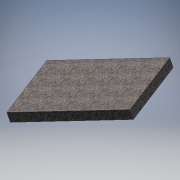
# Autodesk Inventor part: BaseMini
Saved by Autodesk Inventor 2016 (Build 200138000, 138)
## iProperties
Created: 2015-08-01
Part Number: BaseMini
Material: Concrete
Document SubType Name: Modeling
Designer: myhome
Density: 2.40731 g/cm^3
Appearance: Exposed Aggregate - Coarse
Mass: 231102 g
Surface Area: 23200 cm^2
Volume: 96000 cm^3
Author: myhome
Autodesk Inventor part; units mm, degrees
ref_plane "YZ Plane" through (0, 0, 0) normal (1, 0, 0) x (0, 1, 0)
ref_plane "XZ Plane" through (0, 0, 0) normal (0, 1, 0) x (-1, 0, 0)
ref_plane "XY Plane" through (0, 0, 0) normal (0, 0, 1) x (1, 0, 0)
sketch "Sketch5" plane through (0, 0, 0) normal (0, 0, 1) x (1, 0, 0)
  line L0 (0, 0) -> (1200, 0)
  line L1 (1200, 0) -> (1200, 800)
  line L2 (1200, 800) -> (0, 800)
  line L3 (0, 800) -> (0, 0)
  line L4 (1200, 0) -> (1200, 100)
  line L5 (1200, 0) -> (1200, 20)
  line L6 (1200, 20) -> (1200, 120)
  line L7 (0, 0) -> (0, 20) construction
  line L8 (0, 20) -> (0, 120) construction
  line L9 (0, 800) -> (0, 780) construction
  line L10 (0, 680) -> (0, 780) construction
  line L11 (1200, 800) -> (1200, 780) construction
  line L12 (0, 0) -> (0, 100) construction
  line L13 (0, 100) -> (100, 100) construction
  line L14 (100, 100) -> (100, 0) construction
  line L15 (100, 0) -> (0, 0) construction
  circle A0 centre (50, 50) radius 50 construction
  dimension "d12" = 1200
  dimension "d13" = 800
  dimension "d37" = 100
  dimension "d38" = 100
  dimension "d39" = 100
  dimension "d40" = 100
  constraints: 32 end point, 10 point on line, 2 parallel, 2 perpendicular, 1 centre point, 1 collinear, 1 horizontal
  measures "d12" distance of L1.end L2.end
  measures "d13" distance of L0.end L1.end
  measures "d37" distance of L0.start L12.end
  measures "d38" distance of L12.end L13.end
  measures "d39" distance of L13.end L14.end
  measures "d40" diameter of A0
extrude "Extrusion4" add sketch "Sketch5" against normal blind 100
body "Solid2"
